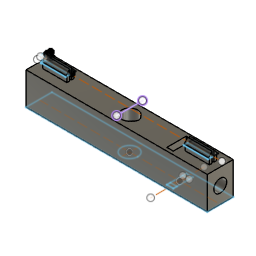
CeilingLightHolder v4 (Autodesk Fusion 360 design; units mm, degrees)
Autodesk Fusion 360 part; units mm, degrees
note: some values were not read from the file. Set by a fixed rule: which sketch regions a step uses.
sketch "Schizzo1" plane through (0, 0, 0) normal (0, 0, 1) x (1, 0, 0)
  line L0 (9, 5) -> (121, 5)
  line L1 (121, 5) -> (121, 21)
  line L2 (121, 21) -> (9, 21)
  line L3 (9, 21) -> (9, 5)
  line L4 (65, 21) -> (65, 5) construction
  line L5 (9, 13) -> (121, 13) construction
  circle A0 centre (65, 13) radius 5
  line L6 (96, 28) -> (96, -5) construction
  line L7 (98, 19) -> (94, 19)
  line L8 (94, 19) -> (94, 7)
  line L9 (94, 7) -> (98, 7)
  line L10 (98, 7) -> (98, 19)
  line L11 (98, 19) -> (94, 7) construction
  line L12 (94, 19) -> (98, 7) construction
  line L13 (94, 7) -> (98, 7)
  line L14 (98, 7) -> (98, 9.2)
  line L15 (98, 9.2) -> (94, 9.2)
  line L16 (94, 9.2) -> (94, 7)
  line L17 (98, 16.8) -> (94, 16.8)
  point P0 (96, 13)
  dimension "d1" = 112
  dimension "d2" = 16
  dimension "d3" = 10
  dimension "d26" = 25
  dimension "d27" = 4
  dimension "d28" = 12
  dimension "d29" = 2.2
  constraint horizontal L0
  constraint vertical L1
  constraint horizontal L2
  constraint vertical L3
  constraint midpoint L2 L4.start
  constraint midpoint L0 L4.end
  constraint midpoint L3 L5.start
  constraint midpoint L1 L5.end
  constraint midpoint L5 A0.centre
  constraint perpendicular L0 L6
  constraint horizontal L7
  constraint perpendicular L7 L8
  constraint parallel L7 L9
  constraint parallel L8 L10
  constraint coincident L11 P0
  constraint coincident L12 P0
  constraint coincident L6 P0
  constraint coincident L5 P0
  constraint horizontal L13
  constraint vertical L14
  constraint horizontal L15
  constraint vertical L16
  constraint coincident L10 L14.end
  constraint symmetric L5 L14.end L17.start
  constraint symmetric L5 L15.end L17.end
  measures "d1" distance of L0.start L0.end
  measures "d2" distance of L0.start L2.end
  measures "d3" diameter of A0
  measures "d26" distance of L1 L6
  measures "d27" distance of L8.end L9.end
  measures "d28" distance of L7.end L8.end
  measures "d29" distance of L8.end L15.end
extrude "Estrusione1" add sketch "Schizzo1" along normal blind 20 contours L0 L1 L2 L3 | L7 L8 L10 L17 | L8 L10 L15 L17 | L8 L9 L10 L13 L14 L15 L16
sketch "Schizzo2" plane through (0, 0, 20) normal (0, 0, 1) x (-1, 0, 0)
  circle A0 centre (-65, -13) radius 5
  line L0 (-9, -21) -> (-9, -5)
  line L1 (-9, -5) -> (-121, -5)
  line L2 (-121, -5) -> (-121, -21)
  line L3 (-121, -21) -> (-9, -21)
  line L4 (-116.5, -10.8) -> (-13.5, -10.8) construction
  line L5 (-13.5, -10.8) -> (-13.5, -15.2) construction
  line L6 (-13.5, -15.2) -> (-116.5, -15.2) construction
  line L7 (-116.5, -15.2) -> (-116.5, -10.8) construction
  line L8 (-116.5, -10.8) -> (-13.5, -15.2) construction
  line L9 (-13.5, -10.8) -> (-116.5, -15.2) construction
  line L10 (-9, -13) -> (-121, -13) construction
  line L11 (-13.5, -15.2) -> (-28.5, -15.2)
  line L12 (-28.5, -15.2) -> (-28.5, -13.6)
  line L13 (-28.5, -13.6) -> (-13.5, -13.6)
  line L14 (-13.5, -13.6) -> (-13.5, -15.2)
  line L15 (-13.5, -10.8) -> (-28.5, -10.8)
  line L16 (-28.5, -12.4) -> (-13.5, -12.4)
  line L17 (-28.5, -10.8) -> (-28.5, -12.4)
  line L18 (-13.5, -15.2) -> (-13.5, -10.8) construction
  line L19 (-65, -21) -> (-65, -5) construction
  line L20 (-13.5, -12.4) -> (-13.5, -10.8)
  line L21 (-116.5, -13.6) -> (-116.5, -15.2)
  line L22 (-101.5, -15.2) -> (-101.5, -13.6)
  line L23 (-101.5, -13.6) -> (-116.5, -13.6)
  line L24 (-116.5, -15.2) -> (-13.5, -15.2) construction
  line L25 (-116.5, -10.8) -> (-101.5, -10.8)
  line L26 (-101.5, -10.8) -> (-101.5, -12.4)
  line L27 (-101.5, -12.4) -> (-116.5, -12.4)
  line L28 (-116.5, -10.8) -> (-116.5, -15.2) construction
  line L29 (-116.5, -12.4) -> (-116.5, -10.8)
  line L30 (-116.5, -15.2) -> (-13.5, -15.2) construction
  line L31 (-116.5, -15.2) -> (-101.5, -15.2)
  point P0 (-65, -13)
  dimension "d6" = 103
  dimension "d7" = 4.4
  dimension "d8" = 15
  dimension "d9" = 1.6
  constraint horizontal L4
  constraint perpendicular L4 L5
  constraint parallel L4 L6
  constraint parallel L5 L7
  constraint coincident L8 P0
  constraint coincident L9 P0
  constraint coincident P0 A0.centre
  constraint midpoint L0 L10.start
  constraint midpoint L2 L10.end
  constraint horizontal L11
  constraint vertical L12
  constraint horizontal L13
  constraint vertical L14
  constraint symmetric L4.end L10 L5.end
  constraint symmetric L5.end L10 L4.end
  constraint symmetric L10 L11.end L15.end
  constraint symmetric L10 L12.end L16.start
  constraint symmetric L10 L13.end L16.end
  constraint midpoint L3 L19.start
  constraint midpoint L1 L19.end
  constraint symmetric L4.end L19 L4.start
  constraint symmetric L5.end L19 L6.end
  constraint symmetric L6.end L19 L5.end
  constraint symmetric L11.end L19 L22.start
  constraint symmetric L12.end L19 L22.end
  constraint symmetric L13.end L19 L21.start
  constraint symmetric L15.end L19 L25.end
  constraint symmetric L16.start L19 L26.end
  constraint symmetric L16.end L19 L27.end
  constraint symmetric L19 L16.end L27.end
  constraint symmetric L19 L4.end L4.start
  measures "d6" distance of L5.end L6.end
  measures "d7" distance of L4.end L5.end
  measures "d8" distance of L5.end L11.end
  measures "d9" distance of L5.end L13.end
extrude "Estrusione2" add sketch "Schizzo2" along normal blind 3.5 contours L11 L12 L13 L14 | L15 L16 L17 L20 | L21 L22 L23 L31 | L25 L26 L27 L29
sketch "Schizzo3" plane through (0, 0, 23.5) normal (0, 0, 1) x (-1, 0, 0)
  line L0 (-13.5, -13.6) -> (-28.5, -13.6)
  line L1 (-28.5, -13.6) -> (-28.5, -15.2)
  line L2 (-28.5, -15.2) -> (-13.5, -15.2)
  line L3 (-13.5, -15.2) -> (-13.5, -13.6)
  line L4 (-10, -13) -> (-122, -13) construction
  line L5 (-65, -21) -> (-65, -5) construction
  line L6 (-28.5, -13.6) -> (-13.5, -13.6)
  line L7 (-13.5, -13.6) -> (-13.5, -16.1)
  line L8 (-13.5, -16.1) -> (-28.5, -16.1)
  line L9 (-28.5, -16.1) -> (-28.5, -13.6)
  line L10 (-28.5, -9.9) -> (-28.5, -12.4)
  line L11 (-13.5, -9.9) -> (-28.5, -9.9)
  line L12 (-13.5, -12.4) -> (-13.5, -9.9)
  line L13 (-28.5, -12.4) -> (-13.5, -12.4)
  line L14 (-116.5, -16.1) -> (-101.5, -16.1)
  line L15 (-116.5, -13.6) -> (-116.5, -16.1)
  line L16 (-101.5, -13.6) -> (-116.5, -13.6)
  line L17 (-101.5, -16.1) -> (-101.5, -13.6)
  line L18 (-101.5, -12.4) -> (-116.5, -12.4)
  line L19 (-116.5, -9.9) -> (-101.5, -9.9)
  line L20 (-101.5, -9.9) -> (-101.5, -12.4)
  line L21 (-116.5, -12.4) -> (-116.5, -9.9)
  line L22 (-65, -21) -> (-65, -5)
  dimension "d12" = 2.5
  constraint horizontal L4
  constraint perpendicular L4 L5
  constraint horizontal L6
  constraint vertical L7
  constraint horizontal L8
  constraint vertical L9
  constraint coincident L0.end L1.start
  constraint collinear L3 L7
  constraint symmetric L4 L0.end L10.end
  constraint symmetric L4 L0.start L12.start
  constraint symmetric L4 L7.end L11.start
  constraint symmetric L4 L8.end L10.start
  constraint symmetric L5 L0.end L16.start
  constraint symmetric L5 L0.start L15.start
  constraint symmetric L5 L7.end L14.start
  constraint symmetric L5 L8.end L14.end
  constraint symmetric L5 L10.start L19.end
  constraint symmetric L5 L10.end L18.start
  constraint symmetric L5 L11.start L19.start
  constraint symmetric L5 L12.start L18.end
  constraint collinear L5 L22
  measures "d12" distance of L0.end L8.end
extrude "Estrusione3" add sketch "Schizzo3" along normal blind 3
sketch "Schizzo5" plane through (13.5, 0, 0) normal (-1, 0, 0) x (0, -1, 0)
  line L0 (-15.2, 20) -> (-13.6, 20)
  line L1 (-13.6, 20) -> (-13.6, 26.5)
  line L2 (-13.6, 26.5) -> (-16.1, 26.5)
  line L3 (-16.1, 26.5) -> (-16.1, 23.5)
  line L4 (-16.1, 23.5) -> (-15.2, 23.5)
  line L5 (-15.2, 23.5) -> (-15.2, 20)
  line L6 (-13.6, 26.5) -> (-16.1, 23.5)
  line L7 (-13.3624, 27.7326) -> (-9.9, 23.5)
  line L8 (-9.9, 23.5) -> (-9.9, 27.7326)
  line L9 (-9.9, 27.7326) -> (-13.3624, 27.7326)
  line L10 (-16.1, 23.5) -> (-15.7, 23.5)
  line L11 (-15.7, 23.5) -> (-15.7, 26.5)
  line L12 (-15.7, 26.5) -> (-16.1, 26.5)
  line L13 (-16.1, 26.5) -> (-16.1, 23.5)
  line L14 (-13, 26.5) -> (-13, 24.5) construction
  line L15 (-10.3, 23.5) -> (-10.3, 26.5)
  line L16 (-9.9, 26.5) -> (-9.9, 23.5)
  line L17 (-10.3, 26.5) -> (-9.9, 26.5)
  line L18 (-9.9, 23.5) -> (-10.3, 23.5)
  line L19 (-16.1, 26.5) -> (-7.5, 26.5) construction
  dimension "d19" = 0.4
  constraint coincident L1.end L2.start
  constraint coincident L3.end L4.start
  constraint vertical L8
  constraint perpendicular L8 L9
  constraint horizontal L10
  constraint vertical L11
  constraint horizontal L12
  constraint vertical L13
  constraint coincident L2 L11.end
  constraint parallel L8 L14
  constraint symmetric L3.end L14 L7.end
  constraint symmetric L10.end L14 L15.start
  constraint symmetric L11.end L14 L15.end
  constraint symmetric L2.end L14 L16.start
  constraint perpendicular L16 L19
  constraint coincident L7.end L8.start
  constraint coincident L14.start L19
  measures "d19" distance of L11 L13
extrude "Estrusione5" cut sketch "Schizzo5" against normal blind 160 contours L2 L6 L11 | L4 L6 L10 L11 | L2 L3 L6 L11 L12 L13 | L7 L8 L9 L15 L17 | L7 L8 L15 L16 L17 | L7 L15 L18
ref_plane "Piano di lavoro1" through (65, 13, 10) normal (0, -1, 0) x (1, 0, 0)
sketch "Schizzo6" plane through (0, 13, 0) normal (0, -1, 0) x (-1, 0, 0)
  line L0 (-9, -20) -> (-121, -20) construction
  line L1 (-121, -20) -> (-121, 0) construction
  line L2 (-121, 0) -> (-9, 0) construction
  line L3 (-9, 0) -> (-9, -20) construction
  line L4 (-65, -20) -> (-65, 0) construction
  line L5 (-9, -10) -> (-121, -10) construction
  line L6 (-65, -20) -> (-75, -10)
  line L7 (-65, -20) -> (-50.8579, -20) construction
  line L8 (-75, -10) -> (-121, -10)
  dimension "d36" = 135
  constraint horizontal L0
  constraint vertical L1
  constraint horizontal L2
  constraint vertical L3
  constraint midpoint L0 L4.start
  constraint midpoint L2 L4.end
  constraint midpoint L3 L5.start
  constraint midpoint L1 L5.end
  constraint horizontal L7
  constraint coincident L5 L6.end
  measures "d36" angle of L6 L7
pipe "Tubo1" cut diameter 8 path "Schizzo6" along L8 L6
extrude "Estrusione6" cut sketch "Schizzo1" along normal blind 10 from surface at 10 contours L8 L10 L15 L17
extrude "Estrusione7" cut sketch "Schizzo1" along normal blind 20 contours L7 L8 L10 L17 | L8 L9 L10 L13 L14 L15 L16
equation "d36 = 180 deg - 45 deg"
